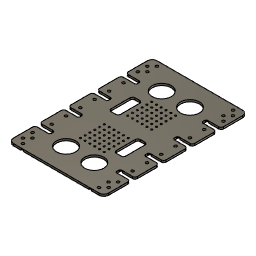
JumperTrunk_BottomPlate_4mm v6 (Autodesk Fusion 360 design; units mm, degrees)
Autodesk Fusion 360 part; units mm, degrees
note: some values were not read from the file. Set by a fixed rule: which sketch regions a step uses.
sketch "Sketch1" plane through (0, 0, 0) normal (0, 1, 0) x (1, 0, 0)
  line L0 (10, 0) -> (189, 0)
  line L1 (189, 300) -> (10, 300)
  circle A0 centre (184, 165) radius 2.75
  circle A1 centre (184, 135) radius 2.75
  circle A2 centre (184, 195) radius 2.75
  circle A3 centre (184, 105) radius 2.75
  arc A4 (10, 300) -> (0, 290) centre (10, 290) ccw
  arc A5 (199, 290) -> (189, 300) centre (189, 290) ccw
  arc A6 (0, 10) -> (10, 0) centre (10, 10) ccw
  arc A7 (189, 0) -> (199, 10) centre (189, 10) ccw
  circle A8 centre (184, 225) radius 2.75
  line L2 (199, 232.541) -> (199, 232)
  line L3 (199, 202) -> (199, 215)
  line L4 (199, 282) -> (199, 290)
  line L5 (194, 175) -> (171, 175)
  line L6 (171, 185) -> (194, 185)
  line L7 (168, 178) -> (168, 182)
  line L8 (194, 115) -> (171, 115)
  line L9 (171, 125) -> (194, 125)
  line L10 (168, 118) -> (168, 122)
  line L11 (0, 290) -> (0, 270)
  line L12 (0, 68.1084) -> (0, 68)
  line L13 (0, 30) -> (0, 10)
  line L14 (199, 10) -> (199, 30)
  line L15 (199, 85) -> (199, 98)
  line L16 (0, 52) -> (0, 52.1084)
  line L17 (0, 112) -> (0, 112.1084)
  line L18 (0, 142) -> (0, 142.1084)
  line L19 (0, 172) -> (0, 172.1084)
  line L20 (0, 202) -> (0, 202.1084)
  line L21 (0, 232) -> (0, 232.1084)
  line L22 (0, 262) -> (0, 262.1084)
  circle A9 centre (15, 105) radius 2.75
  circle A10 centre (15, 135) radius 2.75
  circle A11 centre (15, 165) radius 2.75
  circle A12 centre (15, 195) radius 2.75
  circle A13 centre (15, 225) radius 2.75
  line L23 (5, 115) -> (28, 115)
  line L24 (28, 125) -> (5, 125)
  line L25 (31, 118) -> (31, 122)
  line L26 (28, 185) -> (5, 185)
  line L27 (5, 175) -> (28, 175)
  line L28 (31, 178) -> (31, 182)
  circle A14 centre (10, 280) radius 2.75
  circle A15 centre (20, 270) radius 2.75
  circle A16 centre (20, 290) radius 2.75
  circle A17 centre (20, 30) radius 2.75
  circle A18 centre (10, 20) radius 2.75
  circle A19 centre (20, 10) radius 2.75
  circle A20 centre (179, 10) radius 2.75
  circle A21 centre (189, 20) radius 2.75
  circle A22 centre (179, 30) radius 2.75
  circle A23 centre (179, 270) radius 2.75
  circle A24 centre (189, 280) radius 2.75
  circle A25 centre (179, 290) radius 2.75
  circle A26 centre (70, 90) radius 1.75
  circle A27 centre (129, 210) radius 1.75
  line L29 (199, 270) -> (199, 282)
  line L30 (199, 202) -> (199, 188)
  line L31 (135, 140) -> (145, 140)
  line L32 (150, 135) -> (150, 95)
  line L33 (145, 90) -> (135, 90)
  line L34 (130, 95) -> (130, 135)
  arc A28 (135, 140) -> (130, 135) centre (135, 135) ccw
  arc A29 (150, 135) -> (145, 140) centre (145, 135) ccw
  arc A30 (145, 90) -> (150, 95) centre (145, 95) ccw
  arc A31 (130, 95) -> (135, 90) centre (135, 95) ccw
  line L35 (64, 160) -> (54, 160)
  line L36 (49, 165) -> (49, 205)
  line L37 (54, 210) -> (64, 210)
  line L38 (69, 205) -> (69, 165)
  arc A32 (54, 210) -> (49, 205) centre (54, 205) ccw
  arc A33 (49, 165) -> (54, 160) centre (54, 165) ccw
  arc A34 (64, 160) -> (69, 165) centre (64, 165) ccw
  arc A35 (69, 205) -> (64, 210) centre (64, 205) ccw
  circle A36 centre (70, 50) radius 20
  circle A37 centre (129, 50) radius 20
  circle A38 centre (70, 250) radius 20
  circle A39 centre (129, 250) radius 20
  arc A40 (31, 182) -> (28, 185) centre (28, 182) ccw
  arc A41 (28, 175) -> (31, 178) centre (28, 178) ccw
  arc A42 (31, 122) -> (28, 125) centre (28, 122) ccw
  arc A43 (28, 115) -> (31, 118) centre (28, 118) ccw
  line L39 (0, 112) -> (0, 85)
  arc A44 (171, 125) -> (168, 122) centre (171, 122) ccw
  arc A45 (168, 118) -> (171, 115) centre (171, 118) ccw
  arc A46 (171, 185) -> (168, 182) centre (171, 182) ccw
  arc A47 (168, 178) -> (171, 175) centre (171, 178) ccw
  circle A48 centre (15, 75) radius 2.75
  line L40 (28, 245) -> (5, 245)
  line L41 (5, 235) -> (28, 235)
  arc A49 (28, 235) -> (31, 238) centre (28, 238) ccw
  line L42 (31, 238) -> (31, 242)
  arc A50 (31, 242) -> (28, 245) centre (28, 242) ccw
  line L43 (28, 65) -> (5, 65)
  line L44 (5, 55) -> (28, 55)
  arc A51 (28, 55) -> (31, 58) centre (28, 58) ccw
  line L45 (31, 58) -> (31, 62)
  arc A52 (31, 62) -> (28, 65) centre (28, 62) ccw
  line L46 (0, 30) -> (0, 54.7325)
  line L47 (0, 54.7325) -> (0, 50)
  line L48 (0, 70) -> (0, 85)
  line L49 (0, 112) -> (0, 110)
  line L50 (0, 130) -> (0, 145)
  line L51 (0, 145) -> (0, 170)
  line L52 (0, 190) -> (0, 230)
  line L53 (0, 250) -> (0, 270)
  circle A53 centre (184, 75) radius 2.75
  arc A54 (5, 55) -> (0, 50) centre (5, 50) ccw
  arc A55 (0, 70) -> (5, 65) centre (5, 70) ccw
  arc A56 (5, 115) -> (0, 110) centre (5, 110) ccw
  arc A57 (0, 130) -> (5, 125) centre (5, 130) ccw
  arc A58 (5, 175) -> (0, 170) centre (5, 170) ccw
  arc A59 (0, 190) -> (5, 185) centre (5, 190) ccw
  arc A60 (5, 235) -> (0, 230) centre (5, 230) ccw
  arc A61 (0, 250) -> (5, 245) centre (5, 250) ccw
  line L54 (194, 55) -> (171, 55)
  line L55 (171, 65) -> (194, 65)
  arc A62 (171, 65) -> (168, 62) centre (171, 62) ccw
  arc A63 (168, 58) -> (171, 55) centre (171, 58) ccw
  line L56 (168, 58) -> (168, 62)
  line L57 (171, 245) -> (194, 245)
  line L58 (194, 235) -> (171, 235)
  arc A64 (168, 238) -> (171, 235) centre (171, 238) ccw
  line L59 (168, 238) -> (168, 242)
  arc A65 (171, 245) -> (168, 242) centre (171, 242) ccw
  line L60 (199, 270) -> (199, 250)
  line L61 (199, 230) -> (199, 215)
  line L62 (199, 215) -> (199, 190)
  line L63 (199, 170) -> (199, 130)
  line L64 (199, 110) -> (199, 98)
  line L65 (199, 85) -> (199, 70)
  line L66 (199, 50) -> (199, 30)
  arc A66 (199, 50) -> (194, 55) centre (194, 50) ccw
  arc A67 (194, 65) -> (199, 70) centre (194, 70) ccw
  arc A68 (199, 110) -> (194, 115) centre (194, 110) ccw
  arc A69 (194, 125) -> (199, 130) centre (194, 130) ccw
  arc A70 (199, 170) -> (194, 175) centre (194, 170) ccw
  arc A71 (194, 185) -> (199, 190) centre (194, 190) ccw
  arc A72 (199, 230) -> (194, 235) centre (194, 230) ccw
  arc A73 (194, 245) -> (199, 250) centre (194, 250) ccw
  circle A74 centre (10, 260) radius 2.75
  circle A75 centre (189, 260) radius 2.75
  circle A76 centre (189, 40) radius 2.75
  circle A77 centre (10, 40) radius 2.75
  circle A78 centre (119, 210) radius 1.75
  circle A79 centre (109, 210) radius 1.75
  circle A80 centre (99, 210) radius 1.75
  circle A81 centre (129, 200) radius 1.75
  circle A82 centre (119, 200) radius 1.75
  circle A83 centre (109, 200) radius 1.75
  circle A84 centre (99, 200) radius 1.75
  circle A85 centre (129, 190) radius 1.75
  circle A86 centre (119, 190) radius 1.75
  circle A87 centre (109, 190) radius 1.75
  circle A88 centre (99, 190) radius 1.75
  circle A89 centre (129, 180) radius 1.75
  circle A90 centre (119, 180) radius 1.75
  circle A91 centre (109, 180) radius 1.75
  circle A92 centre (99, 180) radius 1.75
  circle A93 centre (129, 170) radius 1.75
  circle A94 centre (119, 170) radius 1.75
  circle A95 centre (109, 170) radius 1.75
  circle A96 centre (99, 170) radius 1.75
  circle A97 centre (119, 220) radius 1.75
  circle A98 centre (129, 220) radius 1.75
  circle A99 centre (99, 220) radius 1.75
  circle A100 centre (109, 220) radius 1.75
  circle A101 centre (89, 210) radius 1.75
  circle A102 centre (89, 220) radius 1.75
  circle A103 centre (89, 180) radius 1.75
  circle A104 centre (89, 200) radius 1.75
  circle A105 centre (89, 190) radius 1.75
  circle A106 centre (89, 170) radius 1.75
  circle A107 centre (79, 210) radius 1.75
  circle A108 centre (79, 220) radius 1.75
  circle A109 centre (79, 180) radius 1.75
  circle A110 centre (79, 200) radius 1.75
  circle A111 centre (79, 190) radius 1.75
  circle A112 centre (79, 170) radius 1.75
  circle A113 centre (80, 90) radius 1.75
  circle A114 centre (90, 90) radius 1.75
  circle A115 centre (100, 90) radius 1.75
  circle A116 centre (110, 90) radius 1.75
  circle A117 centre (120, 90) radius 1.75
  circle A118 centre (70, 100) radius 1.75
  circle A119 centre (80, 100) radius 1.75
  circle A120 centre (90, 100) radius 1.75
  circle A121 centre (100, 100) radius 1.75
  circle A122 centre (110, 100) radius 1.75
  circle A123 centre (120, 100) radius 1.75
  circle A124 centre (70, 110) radius 1.75
  circle A125 centre (80, 110) radius 1.75
  circle A126 centre (90, 110) radius 1.75
  circle A127 centre (100, 110) radius 1.75
  circle A128 centre (110, 110) radius 1.75
  circle A129 centre (120, 110) radius 1.75
  circle A130 centre (70, 120) radius 1.75
  circle A131 centre (80, 120) radius 1.75
  circle A132 centre (90, 120) radius 1.75
  circle A133 centre (100, 120) radius 1.75
  circle A134 centre (110, 120) radius 1.75
  circle A135 centre (120, 120) radius 1.75
  circle A136 centre (70, 130) radius 1.75
  circle A137 centre (80, 130) radius 1.75
  circle A138 centre (90, 130) radius 1.75
  circle A139 centre (100, 130) radius 1.75
  circle A140 centre (110, 130) radius 1.75
  circle A141 centre (120, 130) radius 1.75
  circle A142 centre (120, 80) radius 1.75
  circle A143 centre (70, 80) radius 1.75
  circle A144 centre (90, 80) radius 1.75
  circle A145 centre (80, 80) radius 1.75
  circle A146 centre (110, 80) radius 1.75
  circle A147 centre (100, 80) radius 1.75
  point P0 (199, 0)
  point P1 (0, 300)
  point P2 (169, 190)
  point P3 (0, 170.1084)
  dimension "d1" = 199
  dimension "d2" = 300
  dimension "d14" = 5.5
  dimension "d21" = 5.5
  dimension "d24" = 5.5
  dimension "d25" = 5.5
  dimension "d39" = 10
  dimension "d40" = 10
  dimension "d41" = 10
  dimension "d42" = 10
  dimension "d53" = 5.5
  dimension "d139" = 5.5
  dimension "d140" = 10
  dimension "d142" = 5.5
  dimension "d144" = 20
  dimension "d145" = 5.5
  dimension "d148" = 0
  dimension "d149" = -260
  dimension "d177" = 3.5
  dimension "d178" = 70
  dimension "d179" = 90
  dimension "d180" = 3.5
  dimension "d181" = 90
  dimension "d198" = 5
  dimension "d199" = 5
  dimension "d202" = 40
  dimension "d203" = 50
  dimension "d205" = 40
  dimension "d207" = 40
  dimension "d208" = 40
  dimension "d211" = 50
  dimension "d212" = 50
  dimension "d232" = 3
  dimension "d233" = 3
  dimension "d234" = 3
  dimension "d235" = 3
  dimension "d246" = 3
  dimension "d247" = 3
  dimension "d248" = 3
  dimension "d249" = 3
  dimension "d258" = 75
  dimension "d259" = 30
  dimension "d260" = 30
  dimension "d261" = 30
  dimension "d262" = 30
  dimension "d263" = 5.5
  dimension "d264" = 15
  dimension "d265" = 30
  dimension "d266" = 3
  dimension "d267" = 3
  dimension "d268" = 3
  dimension "d269" = 3
  dimension "d270" = 75
  dimension "d271" = 30
  dimension "d272" = 30
  dimension "d273" = 30
  dimension "d274" = 30
  dimension "d275" = 5.5
  dimension "d277" = 30
  dimension "d278" = 5
  dimension "d279" = 5
  dimension "d280" = 5
  dimension "d281" = 5
  dimension "d282" = 5
  dimension "d283" = 5
  dimension "d284" = 5
  dimension "d285" = 5
  dimension "d286" = 3
  dimension "d287" = 3
  dimension "d288" = 3
  dimension "d289" = 3
  dimension "d290" = 5
  dimension "d291" = 5
  dimension "d292" = 5
  dimension "d293" = 5
  dimension "d294" = 5
  dimension "d295" = 5
  dimension "d296" = 5
  dimension "d297" = 5
  dimension "d300" = 5.5
  dimension "d301" = 10
  dimension "d302" = 20
  dimension "d303" = 5.5
  dimension "d304" = 10
  dimension "d305" = 20
  dimension "d306" = 5.5
  dimension "d307" = 10
  dimension "d308" = 20
  dimension "d309" = 5.5
  dimension "d310" = 20
  dimension "d315" = -30
  dimension "d316" = -50
  dimension "d321" = 0
  dimension "d322" = 10
  dimension "d329" = 50
  dimension "d330" = 50
  dimension "d333" = 70
  dimension "d334" = 18
  dimension "d335" = 18
  dimension "d338" = 0
  dimension "d339" = -10
  constraint horizontal L0
  constraint vertical L14
  constraint horizontal L1
  constraint vertical L11
  constraint coincident P1 L1
  constraint coincident P1 L11
  constraint tangent L1 A4
  constraint tangent A4 L11
  constraint tangent A5 L14
  constraint tangent L1 A5
  constraint coincident origin L0
  constraint coincident origin L11
  constraint tangent L0 A6
  constraint tangent A6 L11
  constraint coincident P0 L0
  constraint coincident P0 L14
  constraint tangent L0 A7
  constraint tangent A7 L14
  constraint collinear L3 L14
  constraint vertical L2
  constraint coincident P3 L11
  constraint collinear L12 L13
  constraint parallel L11 L22
  constraint coincident L22.end L11
  constraint horizontal L31
  constraint vertical L32
  constraint horizontal L33
  constraint vertical L34
  constraint tangent L31 A28
  constraint tangent L34 A28
  constraint tangent L31 A29
  constraint tangent L32 A29
  constraint equal A28 A29
  constraint tangent L32 A30
  constraint tangent L33 A30
  constraint equal A28 A30
  constraint tangent L33 A31
  constraint tangent L34 A31
  constraint equal A28 A31
  constraint horizontal L35
  constraint vertical L36
  constraint horizontal L37
  constraint vertical L38
  constraint tangent L36 A32
  constraint tangent L37 A32
  constraint tangent L35 A33
  constraint tangent L36 A33
  constraint equal A32 A33
  constraint tangent L35 A34
  constraint tangent L38 A34
  constraint equal A32 A34
  constraint tangent L37 A35
  constraint tangent L38 A35
  constraint equal A32 A35
  constraint tangent L26 A40
  constraint tangent L28 A40
  constraint tangent L28 A41
  constraint tangent L27 A41
  constraint tangent L24 A42
  constraint tangent L25 A42
  constraint tangent L23 A43
  constraint tangent L25 A43
  constraint tangent L10 A44
  constraint tangent L9 A44
  constraint tangent L10 A45
  constraint tangent L8 A45
  constraint tangent L7 A46
  constraint tangent L6 A46
  constraint tangent L7 A47
  constraint tangent L5 A47
  constraint tangent L40 A50
  constraint tangent L42 A50
  constraint tangent A49 L42
  constraint tangent L41 A49
  constraint tangent L43 A52
  constraint tangent L45 A52
  constraint tangent L44 A51
  constraint tangent A51 L45
  constraint parallel L13 L46
  constraint perpendicular L44 L47
  constraint parallel L50 L51
  constraint perpendicular L40 L53
  constraint tangent L47 A54
  constraint coincident L44.start A54.start
  constraint tangent L48 A55
  constraint coincident L43.end A55.end
  constraint tangent L49 A56
  constraint coincident L23.start A56.start
  constraint tangent L50 A57
  constraint coincident L24.end A57.end
  constraint tangent L51 A58
  constraint coincident L27.start A58.start
  constraint tangent L52 A59
  constraint coincident L26.end A59.end
  constraint tangent L52 A60
  constraint coincident L41.start A60.start
  constraint tangent L53 A61
  constraint coincident L40.end A61.end
  constraint tangent A62 L56
  constraint tangent L55 A62
  constraint tangent A63 L56
  constraint tangent L54 A63
  constraint tangent L59 A65
  constraint tangent L57 A65
  constraint tangent A64 L59
  constraint tangent L58 A64
  constraint parallel L29 L60
  constraint parallel L15 L65
  constraint perpendicular L54 L66
  constraint tangent L66 A66
  constraint coincident L54.start A66.end
  constraint tangent L65 A67
  constraint coincident L55.end A67.start
  constraint tangent L64 A68
  constraint coincident L8.start A68.end
  constraint tangent L63 A69
  constraint coincident L9.end A69.start
  constraint tangent L63 A70
  constraint coincident L5.start A70.end
  constraint tangent L62 A71
  constraint coincident L6.end A71.start
  constraint tangent L61 A72
  constraint coincident L58.start A72.end
  constraint tangent L60 A73
  constraint coincident L57.end A73.start
  measures "d1" distance of origin P0
  measures "d2" distance of origin P1
  measures "d14" diameter of A0
  measures "d21" diameter of A1
  measures "d24" diameter of A2
  measures "d25" diameter of A3
  measures "d39" radius of A4
  measures "d40" radius of A5
  measures "d41" radius of A6
  measures "d42" radius of A7
  measures "d53" diameter of A8
  measures "d139" diameter of A14
  measures "d140" distance of L11 A14.centre
  measures "d142" diameter of A15
  measures "d144" distance of L11 A15.centre
  measures "d145" diameter of A16
  measures "d177" diameter of A27
  measures "d178" distance of L3 A27.centre
  measures "d179" distance of L1 A27.centre
  measures "d180" diameter of A26
  measures "d181" distance of L0 A26.centre
  measures "d198" radius of A28
  measures "d199" radius of A32
  measures "d202" diameter of A36
  measures "d203" distance of L0 A36.centre
  measures "d205" diameter of A37
  measures "d207" diameter of A38
  measures "d208" diameter of A39
  measures "d211" distance of L1 A39.centre
  measures "d212" distance of L1 A38.centre
  measures "d232" radius of A40
  measures "d233" radius of A41
  measures "d234" radius of A42
  measures "d235" radius of A43
  measures "d246" radius of A44
  measures "d247" radius of A45
  measures "d248" radius of A46
  measures "d249" radius of A47
  measures "d258" distance of L1 A13.centre
  measures "d259" distance of A12.centre A13.centre
  measures "d260" distance of A11.centre A12.centre
  measures "d261" distance of A10.centre A11.centre
  measures "d262" distance of A9.centre A10.centre
  measures "d263" diameter of A48
  measures "d264" distance of L39 A48.centre
  measures "d265" distance of A9.centre A48.centre
  measures "d266" radius of A50
  measures "d267" radius of A49
  measures "d268" radius of A52
  measures "d269" radius of A51
  measures "d270" distance of L1 A8.centre
  measures "d271" distance of A2.centre A8.centre
  measures "d272" distance of A0.centre A2.centre
  measures "d273" distance of A0.centre A1.centre
  measures "d274" distance of A1.centre A3.centre
  measures "d275" diameter of A53
  measures "d277" distance of A3.centre A53.centre
  measures "d278" radius of A54
  measures "d279" radius of A55
  measures "d280" radius of A56
  measures "d281" radius of A57
  measures "d282" radius of A58
  measures "d283" radius of A59
  measures "d284" radius of A60
  measures "d285" radius of A61
  measures "d286" radius of A62
  measures "d287" radius of A63
  measures "d288" radius of A65
  measures "d289" radius of A64
  measures "d290" radius of A66
  measures "d291" radius of A67
  measures "d292" radius of A68
  measures "d293" radius of A69
  measures "d294" radius of A70
  measures "d295" radius of A71
  measures "d296" radius of A72
  measures "d297" radius of A73
  measures "d300" diameter of A74
  measures "d301" distance of L53 A74.centre
  measures "d302" distance of A14.centre A74.centre
  measures "d303" diameter of A75
  measures "d304" distance of L60 A75.centre
  measures "d305" distance of A24.centre A75.centre
  measures "d306" diameter of A76
  measures "d307" distance of L66 A76.centre
  measures "d308" distance of A21.centre A76.centre
  measures "d309" diameter of A77
  measures "d310" distance of A18.centre A77.centre
  measures "d333" distance of A26.centre L39
  measures "d334" distance of L10 L32
  measures "d335" distance of L28 L36
sketch "Sketch3" plane through (0, 0, 0) normal (0, 1, 0) x (1, 0, 0)
  line L0 (173, 300) -> (168, 300)
  line L1 (168, 300) -> (168, 0)
  line L2 (168, 0) -> (173, 0)
  line L3 (173, 0) -> (173, 300)
  line L4 (31, 300) -> (26, 300)
  line L5 (26, 300) -> (26, 0)
  line L6 (26, 0) -> (31, 0)
  line L7 (31, 0) -> (31, 300)
  line L8 (0, 290) -> (0, 270)
  line L9 (199, 282) -> (199, 290)
  dimension "d152" = 5
  dimension "d154" = 5
  dimension "d155" = 31
  dimension "d215" = 31
  constraint horizontal L0
  constraint vertical L1
  constraint horizontal L2
  constraint vertical L3
  constraint horizontal L4
  constraint vertical L5
  constraint horizontal L6
  constraint vertical L7
  measures "d152" distance of L1 L3
  measures "d154" distance of L5 L7
  measures "d155" distance of L7 L8
  measures "d215" distance of L1 L9
extrude "Extrude15" add sketch "Sketch1" along normal blind 4
extrude "Extrude16" cut sketch "Sketch3" along normal blind 2
